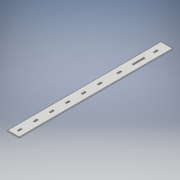
# Autodesk Inventor part: poprz_teownik
Saved by Autodesk Inventor 2017 (Build 210142000, 142)
## iProperties
Created: 2019-10-28
Part Number: poprz_teownik
Material: Ogólny
Document SubType Name: Modeling
Designer: patry
Density: 1 g/cm^3
Appearance: Domyślna
Author: patry
Autodesk Inventor part; units mm, degrees
ref_plane "YZ Plane" through (0, 0, 0) normal (1, 0, 0) x (0, 1, 0)
ref_plane "XZ Plane" through (0, 0, 0) normal (0, 1, 0) x (-1, 0, 0)
ref_plane "XY Plane" through (0, 0, 0) normal (0, 0, 1) x (1, 0, 0)
sketch "Szkic1" plane through (0, 0, 0) normal (0, 0, 1) x (1, 0, 0)
  line L0 (-4.8847, 33.3203) -> (45.1153, 33.3203)
  line L1 (45.1153, 33.3203) -> (45.1153, -636.6797)
  line L2 (45.1153, -636.6797) -> (-4.8847, -636.6797)
  line L3 (-4.8847, -636.6797) -> (-4.8847, 33.3203)
  line L4 (16.8653, -600.6797) -> (22.8653, -600.6797)
  line L5 (22.8653, -600.6797) -> (22.8653, -616.6797)
  line L6 (22.8653, -616.6797) -> (16.8653, -616.6797)
  line L7 (16.8653, -616.6797) -> (16.8653, -600.6797)
  line L8 (16.8653, -530.6797) -> (22.8653, -530.6797)
  line L9 (22.8653, -530.6797) -> (22.8653, -546.6797)
  line L10 (22.8653, -546.6797) -> (16.8653, -546.6797)
  line L11 (16.8653, -546.6797) -> (16.8653, -530.6797)
  line L12 (16.8653, -460.6797) -> (22.8653, -460.6797)
  line L13 (22.8653, -460.6797) -> (22.8653, -476.6797)
  line L14 (22.8653, -476.6797) -> (16.8653, -476.6797)
  line L15 (16.8653, -476.6797) -> (16.8653, -460.6797)
  line L16 (16.8653, -390.6797) -> (22.8653, -390.6797)
  line L17 (22.8653, -390.6797) -> (22.8653, -406.6797)
  line L18 (22.8653, -406.6797) -> (16.8653, -406.6797)
  line L19 (16.8653, -406.6797) -> (16.8653, -390.6797)
  line L20 (16.8653, -320.6797) -> (22.8653, -320.6797)
  line L21 (22.8653, -320.6797) -> (22.8653, -336.6797)
  line L22 (22.8653, -336.6797) -> (16.8653, -336.6797)
  line L23 (16.8653, -336.6797) -> (16.8653, -320.6797)
  line L24 (16.8653, -250.6797) -> (22.8653, -250.6797)
  line L25 (22.8653, -250.6797) -> (22.8653, -266.6797)
  line L26 (22.8653, -266.6797) -> (16.8653, -266.6797)
  line L27 (16.8653, -266.6797) -> (16.8653, -250.6797)
  line L28 (16.8653, -165.6797) -> (22.8653, -165.6797)
  line L29 (22.8653, -165.6797) -> (22.8653, -181.6797)
  line L30 (22.8653, -181.6797) -> (16.8653, -181.6797)
  line L31 (16.8653, -181.6797) -> (16.8653, -165.6797)
  line L32 (22.8653, -21.6797) -> (16.8653, -21.6797)
  line L33 (16.8653, -5.6797) -> (22.8653, -5.6797)
  line L34 (22.8653, -5.6797) -> (22.8653, -21.6797)
  line L35 (16.8653, -21.6797) -> (16.8653, -5.6797)
  line L36 (16.8653, -63.1797) -> (22.8653, -63.1797)
  line L37 (22.8653, -63.1797) -> (22.8653, -114.1797)
  line L38 (22.8653, -114.1797) -> (16.8653, -114.1797)
  line L39 (16.8653, -114.1797) -> (16.8653, -63.1797)
  point P0 (0, 0)
  point P1 (22.8653, -173.6797)
  point P2 (22.8653, -13.6797)
  dimension "d0" = 50
  dimension "d1" = 670
  dimension "d2" = 6
  dimension "d3" = 16
  dimension "d4" = 22.25
  dimension "d5" = 20
  dimension "d8" = 70
  dimension "d13" = 16
  dimension "d14" = 6
  dimension "d16" = 69
  dimension "d17" = 16
  dimension "d18" = 6
  dimension "d19" = 144
  dimension "d20" = 6
  dimension "d21" = 51
  dimension "d22" = 41.5
  constraints: 80 end point, 9 perpendicular, 7 parallel, 3 horizontal, 3 vertical alignment, 2 midpoint, 1 vertical, 40 other
  measures "d0" distance of L1.end L2.end
  measures "d1" distance of L0.end L1.end
  measures "d2" distance of L5.end L6.end
  measures "d3" distance of L4.end L5.end
  measures "d4" distance between parallel lines of L1 L5
  measures "d5" distance between parallel lines of L2 L6
  measures "d8" distance of L4.start L8.start
  measures "d13" distance of L28.end L30.start
  measures "d14" distance of L28.start L28.end
  measures "d16" distance from line of L24 L30.end
  measures "d17" distance of L33.end L32.start
  measures "d18" distance of L35.end L33.end
  measures "d19" distance between parallel lines of L28 L32
  measures "d20" distance of L37.end L38.end
  measures "d21" distance of L36.end L37.end
  measures "d22" distance between parallel lines of L36 L32
extrude "Wyciągnięcie proste1" add sketch "Szkic1" along normal blind 5
